Autodesk Inventor part; units mm, degrees
(part 2 of 2)
sketch "Sketch9" plane through (0, 0, 0) normal (0, -1, 0) x (1, 0, 0)
  line L0 (-3.9405, -13.0371) -> (3.4809, -13.0371) construction
  line L1 (3.4809, -13.0371) -> (3.4809, -15.1214) construction
  line L2 (3.4809, -15.1214) -> (-3.9405, -15.1214) construction
  line L3 (-3.9405, -15.1214) -> (-3.9405, -13.0371) construction
  spline S0 degree 2 poles (-2.9, -15.1182) (-3.1123, -15.1182) (-3.464, -14.9885) (-3.5905, -14.8572) knots 0 0 0 1 2 2 2
  spline S1 degree 2 poles (-3.5905, -14.8572) (-3.7169, -14.7243) (-3.8514, -14.3321) (-3.8514, -14.0776) knots 0 0 0 1 2 2 2
  spline S2 degree 2 poles (-3.8514, -14.0776) (-3.8514, -13.8361) (-3.7153, -13.4536) (-3.5888, -13.3175) knots 0 0 0 1 2 2 2
  spline S3 degree 2 poles (-3.5888, -13.3175) (-3.4673, -13.1862) (-3.1107, -13.0436) (-2.8984, -13.0436) knots 0 0 0 1 2 2 2
  spline S4 degree 2 poles (-2.8984, -13.0436) (-2.7963, -13.0436) (-2.6115, -13.0728) (-2.5273, -13.0987) knots 0 0 0 1 2 2 2
  spline S5 degree 2 poles (-2.5273, -13.0987) (-2.4592, -13.1182) (-2.2939, -13.1895) (-2.2436, -13.2154) knots 0 0 0 1 2 2 2
  line L4 (-2.2436, -13.2154) -> (-2.2436, -13.5363)
  line L5 (-2.2436, -13.5363) -> (-2.2663, -13.5363)
  spline S6 degree 2 poles (-2.2663, -13.5363) (-2.3166, -13.4925) (-2.4219, -13.4131) (-2.5191, -13.3677) knots 0 0 0 1 2 2 2
  spline S7 degree 2 poles (-2.5191, -13.3677) (-2.6002, -13.3272) (-2.8093, -13.2737) (-2.9292, -13.2737) knots 0 0 0 1 2 2 2
  spline S8 degree 2 poles (-2.9292, -13.2737) (-3.2177, -13.2737) (-3.5743, -13.7081) (-3.5743, -14.0695) knots 0 0 0 1 2 2 2
  spline S9 degree 2 poles (-3.5743, -14.0695) (-3.5743, -14.2705) (-3.4802, -14.572) (-3.3911, -14.6757) knots 0 0 0 1 2 2 2
  spline S10 degree 2 poles (-3.3911, -14.6757) (-3.3052, -14.7794) (-3.0621, -14.888) (-2.9097, -14.888) knots 0 0 0 1 2 2 2
  spline S11 degree 2 poles (-2.9097, -14.888) (-2.7979, -14.888) (-2.5743, -14.8556) (-2.4981, -14.8232) knots 0 0 0 1 2 2 2
  line L6 (-2.4981, -14.8232) -> (-2.4981, -14.3062)
  line L7 (-2.4981, -14.3062) -> (-2.9616, -14.3062)
  line L8 (-2.9616, -14.3062) -> (-2.9616, -14.0728)
  line L9 (-2.9616, -14.0728) -> (-2.2355, -14.0728)
  line L10 (-2.2355, -14.0728) -> (-2.2355, -14.9464)
  spline S12 degree 2 poles (-2.2355, -14.9464) (-2.2858, -14.969) (-2.4576, -15.0387) (-2.5305, -15.0598) knots 0 0 0 1 2 2 2
  spline S13 degree 2 poles (-2.5305, -15.0598) (-2.6294, -15.089) (-2.7882, -15.1182) (-2.9, -15.1182) knots 0 0 0 1 2 2 2
  line L11 (-0.5013, -13.0793) -> (-1.1772, -14.1943)
  line L12 (-1.1772, -14.1943) -> (-1.1772, -15.0793)
  line L13 (-1.1772, -15.0793) -> (-1.443, -15.0793)
  line L14 (-1.443, -15.0793) -> (-1.443, -14.2219)
  line L15 (-1.443, -14.2219) -> (-2.1188, -13.0793)
  line L16 (-2.1188, -13.0793) -> (-1.8238, -13.0793)
  line L17 (-1.8238, -13.0793) -> (-1.3084, -13.9593)
  line L18 (-1.3084, -13.9593) -> (-0.7833, -13.0793)
  line L19 (-0.7833, -13.0793) -> (-0.5013, -13.0793)
  line L20 (0.3593, -14.3256) -> (-0.3976, -14.3256)
  line L21 (-0.3976, -14.3256) -> (-0.3976, -14.0825)
  line L22 (-0.3976, -14.0825) -> (0.3593, -14.0825)
  line L23 (0.3593, -14.0825) -> (0.3593, -14.3256)
  spline S14 degree 2 poles (1.1648, -13.2689) (1.0919, -13.2689) (0.9476, -13.3045) (0.8779, -13.3321) knots 0 0 0 1 2 2 2
  spline S15 degree 2 poles (0.8779, -13.3321) (0.8131, -13.3596) (0.7175, -13.418) (0.6802, -13.4439) knots 0 0 0 1 2 2 2
  line L24 (0.6802, -13.4439) -> (0.664, -13.4439)
  line L25 (0.664, -13.4439) -> (0.664, -13.1603)
  spline S16 degree 2 poles (0.664, -13.1603) (0.7515, -13.1133) (1.0514, -13.0371) (1.1859, -13.0371) knots 0 0 0 1 2 2 2
  spline S17 degree 2 poles (1.1859, -13.0371) (1.322, -13.0371) (1.5246, -13.0922) (1.6073, -13.1506) knots 0 0 0 1 2 2 2
  spline S18 degree 2 poles (1.6073, -13.1506) (1.6948, -13.2138) (1.7856, -13.3969) (1.7856, -13.5201) knots 0 0 0 1 2 2 2
  spline S19 degree 2 poles (1.7856, -13.5201) (1.7856, -13.6854) (1.5684, -13.935) (1.416, -13.9674) knots 0 0 0 1 2 2 2
  line L26 (1.416, -13.9674) -> (1.416, -13.9869)
  spline S20 degree 2 poles (1.416, -13.9869) (1.4792, -13.9998) (1.6235, -14.0582) (1.6851, -14.1165) knots 0 0 0 1 2 2 2
  spline S21 degree 2 poles (1.6851, -14.1165) (1.7467, -14.1733) (1.8245, -14.3548) (1.8245, -14.4861) knots 0 0 0 1 2 2 2
  spline S22 degree 2 poles (1.8245, -14.4861) (1.8245, -14.6206) (1.7321, -14.8491) (1.6478, -14.9366) knots 0 0 0 1 2 2 2
  spline S23 degree 2 poles (1.6478, -14.9366) (1.5603, -15.0274) (1.3123, -15.1214) (1.1551, -15.1214) knots 0 0 0 1 2 2 2
  spline S24 degree 2 poles (1.1551, -15.1214) (1.0044, -15.1214) (0.7094, -15.0485) (0.6089, -14.9982) knots 0 0 0 1 2 2 2
  line L27 (0.6089, -14.9982) -> (0.6089, -14.7146)
  line L28 (0.6089, -14.7146) -> (0.6283, -14.7146)
  spline S25 degree 2 poles (0.6283, -14.7146) (0.7126, -14.7762) (0.9979, -14.8896) (1.1389, -14.8896) knots 0 0 0 1 2 2 2
  spline S26 degree 2 poles (1.1389, -14.8896) (1.2215, -14.8896) (1.3868, -14.8378) (1.442, -14.7778) knots 0 0 0 1 2 2 2
  spline S27 degree 2 poles (1.442, -14.7778) (1.4954, -14.7178) (1.5522, -14.5752) (1.5522, -14.4666) knots 0 0 0 1 2 2 2
  spline S28 degree 2 poles (1.5522, -14.4666) (1.5522, -14.358) (1.489, -14.217) (1.4322, -14.1765) knots 0 0 0 1 2 2 2
  spline S29 degree 2 poles (1.4322, -14.1765) (1.3755, -14.136) (1.2215, -14.1052) (1.1308, -14.1052) knots 0 0 0 1 2 2 2
  line L29 (1.1308, -14.1052) -> (1.0173, -14.1052)
  line L30 (1.0173, -14.1052) -> (1.0173, -13.8831)
  line L31 (1.0173, -13.8831) -> (1.1065, -13.8831)
  spline S30 degree 2 poles (1.1065, -13.8831) (1.2864, -13.8831) (1.5133, -13.7113) (1.5133, -13.5476) knots 0 0 0 1 2 2 2
  spline S31 degree 2 poles (1.5133, -13.5476) (1.5133, -13.4715) (1.4549, -13.3629) (1.4079, -13.3305) knots 0 0 0 1 2 2 2
  spline S32 degree 2 poles (1.4079, -13.3305) (1.3577, -13.2964) (1.2345, -13.2689) (1.1648, -13.2689) knots 0 0 0 1 2 2 2
  line L32 (3.2588, -15.0793) -> (2.2831, -15.0793)
  line L33 (2.2831, -15.0793) -> (2.2831, -14.875)
  line L34 (2.2831, -14.875) -> (2.6462, -14.875)
  line L35 (2.6462, -14.875) -> (2.6462, -13.5347)
  line L36 (2.6462, -13.5347) -> (2.2831, -13.5347)
  line L37 (2.2831, -13.5347) -> (2.2831, -13.3515)
  spline S33 degree 2 poles (2.2831, -13.3515) (2.489, -13.3515) (2.6834, -13.2348) (2.6964, -13.0728) knots 0 0 0 1 2 2 2
  line L38 (2.6964, -13.0728) -> (2.9039, -13.0728)
  line L39 (2.9039, -13.0728) -> (2.9039, -14.875)
  line L40 (2.9039, -14.875) -> (3.2588, -14.875)
  line L41 (3.2588, -14.875) -> (3.2588, -15.0793)
  point P0 (0, 0)
  constraints: 2 other
extrude "Extrusion7" add sketch "Sketch9" along normal blind 0.01
sketch "Sketch10" plane through (0, 0, 0) normal (0, -1, 0) x (1, 0, 0)
  line L0 (-16.75, -16.75) -> (16.75, -16.75) projected
  line L1 (16.75, -16.75) -> (16.75, 16.75) projected
  line L2 (-16.75, 16.75) -> (-16.75, -16.75) projected
  point P0 (0, 0)
  point P1 (7.75, -11.25)
  point P2 (5.21, -11.25)
  point P3 (-5.21, -11.25)
  point P4 (-7.75, -11.25)
  dimension "d59" = 2.54
  dimension "d60" = 5.5
  dimension "d61" = 9
  dimension "d62" = 2.54
  dimension "d63" = 5.5
  dimension "d64" = 9
  measures "d59" distance of point (5.21, -11.25) point (7.75, -11.25)
  measures "d60" distance from line of L0 point (7.75, -11.25)
  measures "d61" distance from line of point (7.75, -11.25) L1
  measures "d62" distance of point (-7.75, -11.25) point (-5.21, -11.25)
  measures "d63" distance from line of L0 point (-7.75, -11.25)
  measures "d64" distance from line of L2 point (-7.75, -11.25)
hole "Hole3" at (7.75, 0, -11.25) at (5.21, 0, -11.25) at (-5.21, 0, -11.25) at (-7.75, 0, -11.25) direction (0, 1, 0) diameter 1 depth 8 tip angle 118
sketch "Sketch11" plane through (0, 0, 0) normal (0, -1, 0) x (1, 0, 0)
  circle A0 centre (-5.21, -11.25) radius 0.5 projected
  circle A1 centre (7.75, -11.25) radius 0.5 projected
  circle A2 centre (5.21, -11.25) radius 0.5 projected
  circle A3 centre (-7.75, -11.25) radius 0.5 projected
  line L0 (0.6802, -13.4439) -> (0.664, -13.4439) projected
  line L1 (0.664, -13.4439) -> (0.664, -13.1603) projected
  line L2 (1.416, -13.9674) -> (1.416, -13.9869) projected
  line L3 (0.6089, -14.9982) -> (0.6089, -14.7146) projected
  line L4 (0.6089, -14.7146) -> (0.6283, -14.7146) projected
  line L5 (1.1308, -14.1052) -> (1.0173, -14.1052) projected
  line L6 (1.0173, -14.1052) -> (1.0173, -13.8831) projected
  line L7 (1.0173, -13.8831) -> (1.1065, -13.8831) projected
  line L8 (-1.1772, -14.1943) -> (-1.1772, -15.0793) projected
  line L9 (-1.1772, -15.0793) -> (-1.443, -15.0793) projected
  line L10 (-1.443, -15.0793) -> (-1.443, -14.2219) projected
  line L11 (-1.443, -14.2219) -> (-2.1188, -13.0793) projected
  line L12 (-2.1188, -13.0793) -> (-1.8238, -13.0793) projected
  line L13 (-1.8238, -13.0793) -> (-1.3084, -13.9593) projected
  line L14 (-1.3084, -13.9593) -> (-0.7833, -13.0793) projected
  line L15 (-0.7833, -13.0793) -> (-0.5013, -13.0793) projected
  line L16 (-0.5013, -13.0793) -> (-1.1772, -14.1943) projected
  line L17 (-2.2436, -13.2154) -> (-2.2436, -13.5363) projected
  line L18 (-2.2436, -13.5363) -> (-2.2663, -13.5363) projected
  line L19 (-2.4981, -14.8232) -> (-2.4981, -14.3062) projected
  line L20 (-2.4981, -14.3062) -> (-2.9616, -14.3062) projected
  line L21 (-2.9616, -14.3062) -> (-2.9616, -14.0728) projected
  line L22 (-2.9616, -14.0728) -> (-2.2355, -14.0728) projected
  line L23 (-2.2355, -14.0728) -> (-2.2355, -14.9464) projected
  line L24 (-0.3976, -14.3256) -> (-0.3976, -14.0825) projected
  line L25 (-0.3976, -14.0825) -> (0.3593, -14.0825) projected
  line L26 (0.3593, -14.0825) -> (0.3593, -14.3256) projected
  line L27 (0.3593, -14.3256) -> (-0.3976, -14.3256) projected
  line L28 (2.2831, -15.0793) -> (2.2831, -14.875) projected
  line L29 (2.2831, -14.875) -> (2.6462, -14.875) projected
  line L30 (2.6462, -14.875) -> (2.6462, -13.5347) projected
  line L31 (2.6462, -13.5347) -> (2.2831, -13.5347) projected
  line L32 (2.2831, -13.5347) -> (2.2831, -13.3515) projected
  line L33 (2.6964, -13.0728) -> (2.9039, -13.0728) projected
  line L34 (2.9039, -13.0728) -> (2.9039, -14.875) projected
  line L35 (2.9039, -14.875) -> (3.2588, -14.875) projected
  line L36 (3.2588, -14.875) -> (3.2588, -15.0793) projected
  line L37 (3.2588, -15.0793) -> (2.2831, -15.0793) projected
  circle A4 centre (-12.75, 2.55) radius 0.5 projected
  circle A5 centre (-12.75, -2.53) radius 0.5 projected
  circle A6 centre (-12.75, -5.07) radius 0.5 projected
  circle A7 centre (-12.75, 0.01) radius 0.5 projected
  circle A8 centre (-12.75, 5.09) radius 0.5 projected
  circle A9 centre (12.75, 2.55) radius 0.5 projected
  circle A10 centre (12.75, -2.53) radius 0.5 projected
  circle A11 centre (12.75, -5.07) radius 0.5 projected
  circle A12 centre (12.75, 0.01) radius 0.5 projected
  circle A13 centre (12.75, 5.09) radius 0.5 projected
  circle A14 centre (-12.4997, -12.3836) radius 2.5 projected
  circle A15 centre (12.5, 12.5) radius 2.5 projected
  circle A16 centre (12.5, -12.5) radius 2.5 projected
  circle A17 centre (-12.4997, 12.6164) radius 2.5 projected
  line L38 (16.75, 16.75) -> (-16.75, 16.75) projected
  line L39 (-16.75, 16.75) -> (-16.75, -16.75) projected
  line L40 (-16.75, -16.75) -> (16.75, -16.75) projected
  line L41 (16.75, -16.75) -> (16.75, 16.75) projected
  circle A18 centre (-7.75, -11.25) radius 1
  circle A19 centre (-5.21, -11.25) radius 0.5 projected
  circle A20 centre (-5.21, -11.25) radius 1
  circle A21 centre (5.21, -11.25) radius 0.5 projected
  circle A22 centre (5.21, -11.25) radius 1
  circle A23 centre (7.75, -11.25) radius 0.5 projected
  circle A24 centre (7.75, -11.25) radius 1
  point P0 (0, 0)
  dimension "d72" = 2
  dimension "d73" = 2
  dimension "d74" = 2
  dimension "d75" = 2
  constraints: 4 centre point, 4 coincident, 34 other
  measures "d72" diameter of A18
  measures "d73" diameter of A20
  measures "d74" diameter of A22
  measures "d75" diameter of A24
extrude "Extrusion8" add sketch "Sketch11" along normal blind 0.01 contours A18 | A20 | A22 | A24
sketch "Sketch12" plane through (0, 1.65, 0) normal (0, 1, 0) x (1, 0, 0)
  circle A0 centre (-5.21, 11.25) radius 0.5 projected
  circle A1 centre (7.75, 11.25) radius 0.5 projected
  circle A2 centre (5.21, 11.25) radius 0.5 projected
  circle A3 centre (-7.75, 11.25) radius 0.5 projected
  line L0 (-11.1, 6.49) -> (-11.1, -6.51) projected
  line L1 (-11.1, -6.51) -> (-14.4, -6.51) projected
  line L2 (-14.4, -6.51) -> (-14.4, 6.49) projected
  line L3 (-14.4, 6.49) -> (-11.1, 6.49) projected
  line L4 (-16.75, -16.75) -> (16.75, -16.75) projected
  line L5 (16.75, -16.75) -> (16.75, 16.75) projected
  line L6 (16.75, 16.75) -> (-16.75, 16.75) projected
  line L7 (-16.75, 16.75) -> (-16.75, -16.75) projected
  circle A4 centre (12.5, -12.5) radius 2.5 projected
  circle A5 centre (-12.4997, 12.3836) radius 2.5 projected
  circle A6 centre (-12.4997, -12.6164) radius 2.5 projected
  circle A7 centre (12.5, 12.5) radius 2.5 projected
  line L8 (11.1, -6.51) -> (11.1, 6.49) projected
  line L9 (11.1, 6.49) -> (14.4, 6.49) projected
  line L10 (14.4, 6.49) -> (14.4, -6.51) projected
  line L11 (14.4, -6.51) -> (11.1, -6.51) projected
  line L12 (-14.9849, -7.5616) -> (-15.1854, -7.5616) projected
  line L13 (-15.1854, -7.5616) -> (-15.1854, -7.5484) projected
  line L14 (-15.8682, -7.5494) -> (-15.8682, -7.5616) projected
  line L15 (-15.8682, -7.5616) -> (-16.0667, -7.5616) projected
  line L16 (-16.1518, -5.1021) -> (-16.1518, -4.9228) projected
  line L17 (-16.1518, -4.9228) -> (-14.9018, -4.4923) projected
  line L18 (-14.9018, -4.4923) -> (-14.9018, -4.6706) projected
  line L19 (-14.9018, -4.6706) -> (-15.9401, -5.017) projected
  line L20 (-15.9401, -5.017) -> (-14.9018, -5.3635) projected
  line L21 (-14.9018, -5.3635) -> (-14.9018, -5.5326) projected
  line L22 (-14.9018, -5.5326) -> (-16.1518, -5.1021) projected
  line L23 (-16.0768, -2.1321) -> (-15.8682, -2.1321) projected
  line L24 (-15.8682, -2.1321) -> (-15.8682, -2.1443) projected
  line L25 (-14.9606, -2.9334) -> (-15.1591, -2.9334) projected
  line L26 (-15.1591, -2.9334) -> (-15.1591, -2.9212) projected
  line L27 (-16.0768, 0.3) -> (-15.8682, 0.3) projected
  line L28 (-15.8682, 0.3) -> (-15.8682, 0.2879) projected
  line L29 (-14.9606, -0.5012) -> (-15.1591, -0.5012) projected
  line L30 (-15.1591, -0.5012) -> (-15.1591, -0.4891) projected
  line L31 (-15.6818, 2.9216) -> (-14.9018, 2.9216) projected
  line L32 (-14.9018, 2.9216) -> (-14.9018, 2.7555) projected
  line L33 (-14.9018, 2.7555) -> (-15.6818, 2.7555) projected
  line L34 (-15.6858, 2.1831) -> (-14.9018, 2.1831) projected
  line L35 (-14.9018, 2.1831) -> (-14.9018, 2.017) projected
  line L36 (-14.9018, 2.017) -> (-15.6818, 2.017) projected
  line L37 (-16.1518, 5.5381) -> (-16.1518, 5.8258) projected
  line L38 (-16.1518, 5.8258) -> (-14.9018, 5.8258) projected
  line L39 (-14.9018, 5.8258) -> (-14.9018, 5.5411) projected
  line L40 (-14.9869, 7.1872) -> (-15.1875, 7.1872) projected
  line L41 (-15.1875, 7.1872) -> (-15.1875, 7.2014) projected
  line L42 (-15.9918, 7.3462) -> (-15.6686, 7.3462) projected
  line L43 (-15.6686, 7.3462) -> (-15.6686, 7.6359) projected
  line L44 (-15.6686, 7.6359) -> (-15.5228, 7.6359) projected
  line L45 (-15.5228, 7.6359) -> (-15.5228, 7.1821) projected
  line L46 (-15.5228, 7.1821) -> (-16.0687, 7.1821) projected
  line L47 (16.18, 7.1148) -> (16.18, 6.8271) projected
  line L48 (16.18, 6.8271) -> (14.93, 6.8271) projected
  line L49 (14.93, 6.8271) -> (14.93, 7.1118) projected
  line L50 (15.015, 5.4657) -> (15.2156, 5.4657) projected
  line L51 (15.2156, 5.4657) -> (15.2156, 5.4515) projected
  line L52 (16.0199, 5.3067) -> (15.6968, 5.3067) projected
  line L53 (15.6968, 5.3067) -> (15.6968, 5.017) projected
  line L54 (15.6968, 5.017) -> (15.5509, 5.017) projected
  line L55 (15.5509, 5.017) -> (15.5509, 5.4708) projected
  line L56 (15.5509, 5.4708) -> (16.0969, 5.4708) projected
  line L57 (16.18, 3.1166) -> (16.18, 2.8289) projected
  line L58 (16.18, 2.8289) -> (14.93, 2.8289) projected
  line L59 (14.93, 2.8289) -> (14.93, 3.1136) projected
  line L60 (16.18, 1.0097) -> (14.93, 1.0097) projected
  line L61 (14.93, 1.0097) -> (14.93, 1.1758) projected
  line L62 (14.93, 1.1758) -> (16.0321, 1.1758) projected
  line L63 (16.0321, 1.1758) -> (16.0321, 1.7339) projected
  line L64 (16.0321, 1.7339) -> (16.18, 1.7339) projected
  line L65 (16.18, 1.7339) -> (16.18, 1.0097) projected
  line L66 (16.18, -2.8345) -> (16.0523, -2.8345) projected
  line L67 (16.0523, -2.8345) -> (16.0523, -2.6076) projected
  line L68 (16.0523, -2.6076) -> (15.2146, -2.6076) projected
  line L69 (15.2146, -2.6076) -> (15.2146, -2.8345) projected
  line L70 (15.2146, -2.8345) -> (15.1001, -2.8345) projected
  line L71 (14.9259, -2.5762) -> (14.9259, -2.4466) projected
  line L72 (14.9259, -2.4466) -> (16.0523, -2.4466) projected
  line L73 (16.0523, -2.4466) -> (16.0523, -2.2247) projected
  line L74 (16.0523, -2.2247) -> (16.18, -2.2247) projected
  line L75 (16.18, -2.2247) -> (16.18, -2.8345) projected
  line L76 (15.013, -4.5465) -> (15.2136, -4.5465) projected
  line L77 (15.2136, -4.5465) -> (15.2136, -4.5596) projected
  line L78 (15.8963, -4.5586) -> (15.8963, -4.5465) projected
  line L79 (15.8963, -4.5465) -> (16.0949, -4.5465) projected
  line L80 (16.18, -7.0059) -> (16.18, -7.1852) projected
  line L81 (16.18, -7.1852) -> (14.93, -7.6157) projected
  line L82 (14.93, -7.6157) -> (14.93, -7.4375) projected
  line L83 (14.93, -7.4375) -> (15.9682, -7.091) projected
  line L84 (15.9682, -7.091) -> (14.93, -6.7446) projected
  line L85 (14.93, -6.7446) -> (14.93, -6.5754) projected
  line L86 (14.93, -6.5754) -> (16.18, -7.0059) projected
  line L87 (15.013, -5.5787) -> (15.2136, -5.5787) projected
  line L88 (15.2136, -5.5787) -> (15.2136, -5.5918) projected
  line L89 (15.8963, -5.5908) -> (15.8963, -5.5787) projected
  line L90 (15.8963, -5.5787) -> (16.0949, -5.5787) projected
  line L91 (16.105, -3.9164) -> (15.8963, -3.9164) projected
  line L92 (15.8963, -3.9164) -> (15.8963, -3.9042) projected
  line L93 (14.9887, -3.1151) -> (15.1873, -3.1151) projected
  line L94 (15.1873, -3.1151) -> (15.1873, -3.1273) projected
  line L95 (16.105, -1.4843) -> (15.8963, -1.4843) projected
  line L96 (15.8963, -1.4843) -> (15.8963, -1.4721) projected
  line L97 (14.9887, -0.683) -> (15.1873, -0.683) projected
  line L98 (15.1873, -0.683) -> (15.1873, -0.6952) projected
  line L99 (14.93, 1.8646) -> (14.93, 2.6466) projected
  line L100 (14.93, 2.6466) -> (15.0779, 2.6466) projected
  line L101 (15.0779, 2.6466) -> (15.0779, 2.0307) projected
  line L102 (15.0779, 2.0307) -> (15.4202, 2.0307) projected
  line L103 (15.4202, 2.0307) -> (15.4202, 2.6051) projected
  line L104 (15.4202, 2.6051) -> (15.5681, 2.6051) projected
  line L105 (15.5681, 2.6051) -> (15.5681, 2.0307) projected
  line L106 (15.5681, 2.0307) -> (16.0321, 2.0307) projected
  line L107 (16.0321, 2.0307) -> (16.0321, 2.6466) projected
  line L108 (16.0321, 2.6466) -> (16.18, 2.6466) projected
  line L109 (16.18, 2.6466) -> (16.18, 1.8646) projected
  line L110 (16.18, 1.8646) -> (14.93, 1.8646) projected
  line L111 (16.18, 6.3875) -> (15.1022, 5.8344) projected
  line L112 (15.1022, 5.8344) -> (16.18, 5.8344) projected
  line L113 (16.18, 5.8344) -> (16.18, 5.6794) projected
  line L114 (16.18, 5.6794) -> (14.93, 5.6794) projected
  line L115 (14.93, 5.6794) -> (14.93, 5.9155) projected
  line L116 (14.93, 5.9155) -> (15.9196, 6.4189) projected
  line L117 (15.9196, 6.4189) -> (14.93, 6.4189) projected
  line L118 (14.93, 6.4189) -> (14.93, 6.5739) projected
  line L119 (14.93, 6.5739) -> (16.18, 6.5739) projected
  line L120 (16.18, 6.5739) -> (16.18, 6.3875) projected
  line L121 (-16.1518, 6.2654) -> (-15.074, 6.8185) projected
  line L122 (-15.074, 6.8185) -> (-16.1518, 6.8185) projected
  line L123 (-16.1518, 6.8185) -> (-16.1518, 6.9734) projected
  line L124 (-16.1518, 6.9734) -> (-14.9018, 6.9734) projected
  line L125 (-14.9018, 6.9734) -> (-14.9018, 6.7374) projected
  line L126 (-14.9018, 6.7374) -> (-15.8915, 6.234) projected
  line L127 (-15.8915, 6.234) -> (-14.9018, 6.234) projected
  line L128 (-14.9018, 6.234) -> (-14.9018, 6.079) projected
  line L129 (-14.9018, 6.079) -> (-16.1518, 6.079) projected
  line L130 (-16.1518, 6.079) -> (-16.1518, 6.2654) projected
  line L131 (-15.0497, 1.4872) -> (-15.0497, 1.9066) projected
  line L132 (-15.0497, 1.9066) -> (-14.9018, 1.9066) projected
  line L133 (-14.9018, 1.9066) -> (-14.9018, 0.9017) projected
  line L134 (-14.9018, 0.9017) -> (-15.0497, 0.9017) projected
  line L135 (-15.0497, 0.9017) -> (-15.0497, 1.3211) projected
  line L136 (-15.0497, 1.3211) -> (-16.1518, 1.3211) projected
  line L137 (-16.1518, 1.3211) -> (-16.1518, 1.4872) projected
  line L138 (-16.1518, 1.4872) -> (-15.0497, 1.4872) projected
  line L139 (-16.1518, -0.6836) -> (-15.9745, -0.6836) projected
  line L140 (-15.1287, -0.719) -> (-15.1287, -0.7099) projected
  line L141 (-15.1287, -0.7099) -> (-14.9504, -0.7099) projected
  line L142 (-16.007, -0.8406) -> (-16.007, -1.4544) projected
  line L143 (-16.007, -1.4544) -> (-16.1518, -1.4544) projected
  line L144 (-16.1518, -1.4544) -> (-16.1518, -0.6836) projected
  line L145 (-15.1297, -3.1501) -> (-15.1297, -3.14) projected
  line L146 (-15.1297, -3.14) -> (-14.9525, -3.14) projected
  line L147 (-15.4569, -3.61) -> (-15.4691, -3.61) projected
  line L148 (-16.1012, -3.1056) -> (-15.9239, -3.1056) projected
  line L149 (-15.9239, -3.1056) -> (-15.9239, -3.1177) projected
  line L150 (-15.543, -3.4317) -> (-15.543, -3.3608) projected
  line L151 (-15.543, -3.3608) -> (-15.4042, -3.3608) projected
  line L152 (-15.4042, -3.3608) -> (-15.4042, -3.4165) projected
  line L153 (-14.9849, -6.5294) -> (-15.1854, -6.5294) projected
  line L154 (-15.1854, -6.5294) -> (-15.1854, -6.5162) projected
  line L155 (-15.8682, -6.5172) -> (-15.8682, -6.5294) projected
  line L156 (-15.8682, -6.5294) -> (-16.0667, -6.5294) projected
  circle A8 centre (7.75, 11.25) radius 1
  circle A9 centre (5.21, 11.25) radius 1
  circle A10 centre (-5.21, 11.25) radius 1
  circle A11 centre (-7.75, 11.25) radius 1
  point P0 (0, 0)
  dimension "d78" = 2
  dimension "d79" = 2
  dimension "d80" = 2
  dimension "d81" = 2
  constraints: 4 centre point, 4 coincident, 219 other
  measures "d78" diameter of A8
  measures "d79" diameter of A9
  measures "d80" diameter of A10
  measures "d81" diameter of A11
extrude "Extrusion9" add sketch "Sketch12" along normal blind 0.01 contours A8 | A9 | A10 | A11
mirror "Mirror4" about plane through (0, 0, 0) normal (0, 0, 1) of "Hole3", "Extrusion9", "Extrusion8"
sketch "Sketch13" plane through (0, 1.65, 0) normal (0, 1, 0) x (1, 0, 0)
  line L0 (-8, 8) -> (8, 8)
  line L1 (8, 8) -> (8, -8)
  line L2 (8, -8) -> (-8, -8)
  line L3 (-8, -8) -> (-8, 8)
  line L4 (-8, 8) -> (8, -8) construction
  line L5 (8, 8) -> (-8, -8) construction
  line L6 (0, 10) -> (0, -10) construction
  line L7 (-2.15, 10) -> (-2.15, -10)
  line L8 (2.15, -10) -> (2.15, 10)
  arc A0 (2.15, 10) -> (-2.15, 10) centre (0, 10) ccw
  arc A1 (-2.15, -10) -> (2.15, -10) centre (0, -10) ccw
  point P0 (0, 0)
  dimension "d84" = 16
  dimension "d85" = 16
  dimension "d86" = 10
  dimension "d87" = 4.3
  constraints: 20 end point, 4 point on circle, 4 tangent, 3 midpoint, 3 parallel, 2 centre point, 1 horizontal, 1 perpendicular, 1 vertical
  measures "d84" distance of L1.end L2.end
  measures "d85" distance of L0.end L1.end
  measures "d86" distance of point (0, 0) L6.end
  measures "d87" diameter of A1
extrude "Extrusion10" add sketch "Sketch13" along normal blind 7
sketch "Sketch14" plane through (0, 8.65, 0) normal (0, 1, 0) x (1, 0, 0)
  circle A0 centre (0, 0) radius 7.9
  dimension "d90" = 15.8
  constraints: 1 centre point, 1 coincident
  measures "d90" diameter of A0
extrude "Extrusion11" add sketch "Sketch14" along normal blind 3
sketch "Sketch15" plane through (0, 8.65, 0) normal (0, 1, 0) x (1, 0, 0)
  circle A0 centre (0, 0) radius 7.9 projected
  line L0 (2.15, -8) -> (8, -8) projected
  line L1 (8, -8) -> (8, 8) projected
  line L2 (8, 8) -> (2.15, 8) projected
  line L3 (2.15, 8) -> (2.15, 10) projected
  arc A1 (2.15, 10) -> (-2.15, 10) centre (0, 10) ccw projected
  line L4 (-2.15, 10) -> (-2.15, 8) projected
  line L5 (-2.15, 8) -> (-8, 8) projected
  line L6 (-8, 8) -> (-8, -8) projected
  line L7 (-8, -8) -> (-2.15, -8) projected
  line L8 (-2.15, -8) -> (-2.15, -10) projected
  arc A2 (-2.15, -10) -> (2.15, -10) centre (0, -10) ccw projected
  line L9 (2.15, -10) -> (2.15, -8) projected
  constraints: 2 coincident
hole "Hole4" at (0, 8.65, 10) at (0, 8.65, -10) direction (0, -1, 0) diameter 1 end through all
sketch "Sketch16" plane through (-8, 1.65, -8) normal (-1, 0, 0) x (0, 0, 1)
  line L0 (9.75, 2.3488) -> (6.25, 2.3488)
  line L1 (6.25, 2.3488) -> (6.25, 9.4579)
  line L2 (6.25, 9.4579) -> (9.75, 9.4579)
  line L3 (9.75, 9.4579) -> (9.75, 2.3488)
  line L4 (9.75, 2.3488) -> (6.25, 9.4579) construction
  line L5 (6.25, 2.3488) -> (9.75, 9.4579) construction
  point P0 (8, -1.65)
  point P1 (8, 5.9034)
  dimension "d100" = 3.5
  constraints: 12 end point, 2 midpoint, 2 parallel, 1 horizontal, 1 perpendicular
  measures "d100" distance of L1.end L2.end
extrude "Extrusion12" add sketch "Sketch16" along normal blind 0.9 and the other way blind 1.5
fillet "Fillet1" radius 0.02 2 edges at (0.8805, 8.65, -7.8508) (0.8805, 8.65, 7.8508)
fillet "Fillet2" radius 0.02 39 edges at (-5.075, 8.65, -8) (0, 8.65, -12.15) (2.15, 8.65, -9) (-2.15, 8.65, -9) (5.075, 8.65, -8) (8, 8.65, 0) (-8, 8.65, -4.875) (-8, 8.65, 4.875) (-8, 5.15, -8) (-2.15, 5.15, -8) (2.15, 5.15, -8) (8, 5.15, -8) (-8.9, 7.5534, -1.75) (-8.9, 7.5534, 1.75) (-8.9, 3.9988, 0) (-8.45, 3.9988, -1.75) (-8, 6.3244, -1.75) (-8.3019, 11.1079, -1.75) (-8.3019, 11.1079, 1.75) (-7.9, 11.1079, 0) (-8.45, 3.9988, 1.75) (-8, 3.9988, 0) (-8, 6.3244, 1.75) (-7.7097, 8.6559, 1.75) (-7.8621, 8.65, 1.75) (-7.7037, 9.8889, 1.75) (-7.7097, 8.6559, -1.75) (-7.8621, 8.65, -1.75) (-7.7037, 9.8889, -1.75) (-5.075, 8.65, 8) (-8, 5.15, 8) (-2.15, 5.15, 8) (0, 8.65, 12.15) (2.15, 8.65, 9) (-2.15, 8.65, 9) (5.075, 8.65, 8) (2.15, 5.15, 8) (8, 5.15, 8) (-7.9, 11.65, 0)
sketch "Sketch17" plane through (0, 11.65, 0) normal (0, 1, 0) x (1, 0, 0)
  circle A0 centre (0, 0) radius 5.74
  circle A1 centre (0, 0) radius 7.88 projected
  dimension "d107" = 2.14
  constraints: 1 centre point, 1 coincident
  measures "d107" radial gap between concentric circles of A1 A0
extrude "Extrusion13" cut sketch "Sketch17" against normal up to surface (10 mm away) contours A0
sketch "Sketch18" plane through (0, 1.65, 0) normal (0, 1, 0) x (1, 0, 0)
  line L0 (-7.98, -1.77) -> (-7.7197, -1.77) projected
  line L1 (-7.98, -7.98) -> (-7.98, -1.77) projected
  line L2 (-2.17, -7.98) -> (-7.98, -7.98) projected
  arc A0 (-2.13, -8.02) -> (-2.17, -7.98) centre (-2.17, -8.02) ccw projected
  line L3 (-2.13, -10) -> (-2.13, -8.02) projected
  arc A1 (-2.13, -10) -> (2.13, -10) centre (0, -10) ccw projected
  line L4 (2.13, -8.02) -> (2.13, -10) projected
  arc A2 (2.17, -7.98) -> (2.13, -8.02) centre (2.17, -8.02) ccw projected
  line L5 (7.98, -7.98) -> (2.17, -7.98) projected
  line L6 (7.98, 7.98) -> (7.98, -7.98) projected
  line L7 (2.17, 7.98) -> (7.98, 7.98) projected
  arc A3 (2.13, 8.02) -> (2.17, 7.98) centre (2.17, 8.02) ccw projected
  line L8 (2.13, 10) -> (2.13, 8.02) projected
  arc A4 (2.13, 10) -> (-2.13, 10) centre (0, 10) ccw projected
  line L9 (-2.13, 8.02) -> (-2.13, 10) projected
  arc A5 (-2.17, 7.98) -> (-2.13, 8.02) centre (-2.17, 8.02) ccw projected
  line L10 (-7.98, 7.98) -> (-2.17, 7.98) projected
  line L11 (-7.98, 1.77) -> (-7.98, 7.98) projected
  line L12 (-7.7197, 1.77) -> (-7.98, 1.77) projected
  arc A6 (-7.7197, -1.77) -> (-7.7197, 1.77) centre (0, 0) ccw projected
  circle A7 centre (0, -10) radius 0.5 projected
  circle A8 centre (0, 10) radius 0.5 projected
  circle A9 centre (0, 0) radius 5.74 projected
  circle A10 centre (0, 0) radius 7.88 projected
  line L13 (6.98, 6.98) -> (-6.98, 6.98)
  line L14 (-6.98, 6.98) -> (-6.98, -6.98)
  line L15 (-6.98, -6.98) -> (6.98, -6.98)
  line L16 (6.98, -6.98) -> (6.98, 6.98)
  line L17 (6.98, 6.98) -> (-6.98, -6.98) construction
  line L18 (-6.98, 6.98) -> (6.98, -6.98) construction
  dimension "d111" = 1
  dimension "d112" = 1
  constraints: 12 end point, 2 midpoint, 2 parallel, 1 horizontal, 1 perpendicular
  measures "d111" distance between parallel lines of L1 L14
  measures "d112" distance between parallel lines of L2 L15
extrude "Extrusion14" cut sketch "Sketch18" along normal blind 6.4 contours L14 A10 L15 A6 | A6 L15 L14 | L14 A10 L13 L16 L15 | L15 A10 L16 A6 | A6 L16 L15 | L14 A6 L13 A10 | L14 L13 A6 | L16 A10 L13 A6 | A6 L13 L16
sketch "Sketch19" plane through (5.21, 1.66, 11.25) normal (0, 1, 0) x (1, 0, 0)
  circle A0 centre (0, 0) radius 0.5 projected
  circle A1 centre (0, 0) radius 1 projected
  point P0 (-5.21, 11.25)
  constraints: 1 coincident
sketch "Sketch20" plane through (7.75, 1.66, 11.25) normal (0, 1, 0) x (1, 0, 0)
  circle A0 centre (0, 0) radius 1 projected
  point P0 (-7.75, 11.25)
  constraints: 1 coincident
thread "Thread1" size "M12x1.75" class "6H" standard "ANSI Metric M Profile" full length
ref_plane "Work Plane1" through (0, 0, 0) normal (1, 0, 0) x (0, 1, 0)
body "Solid1"
